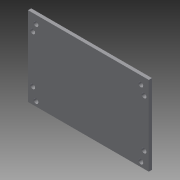
# Autodesk Inventor part: circuit_plate
Saved by Autodesk Inventor 2013 (Build 170138000, 138)
## iProperties
Created: 2014-05-23
Part Number: circuit_plate
Material: 一般
Document SubType Name: Modeling
Designer: andou
Density: 1 g/cm^3
Author: andou
Autodesk Inventor part; units mm, degrees
ref_plane "YZ Plane" through (0, 0, 0) normal (1, 0, 0) x (0, 1, 0)
ref_plane "XZ Plane" through (0, 0, 0) normal (0, 1, 0) x (-1, 0, 0)
ref_plane "XY Plane" through (0, 0, 0) normal (0, 0, 1) x (1, 0, 0)
sketch "スケッチ1" plane through (0, 0, 0) normal (0, 1, 0) x (-1, 0, 0)
  line L0 (-38, 35) -> (38, 35)
  line L1 (38, 35) -> (38, -15)
  line L2 (38, -15) -> (-38, -15)
  line L3 (-38, -15) -> (-38, 35)
  point P0 (0, 0)
  dimension "d0" = 76
  dimension "d3" = 50
  dimension "d4" = 35
  dimension "d5" = 38
  constraints: 8 end point, 2 parallel, 1 horizontal, 1 perpendicular
  measures "d0" distance of L0.start L0.end
  measures "d3" distance of L2.end L0.start
  measures "d4" distance from line of L0 point (0, 0)
  measures "d5" distance from line of L3 point (0, 0)
extrude "押し出し1" add sketch "スケッチ1" along normal blind 2
sketch "スケッチ2" plane through (0, 2, 0) normal (0, 1, 0) x (1, 0, 0)
  line L0 (-38, -35) -> (38, -35) projected
  line L1 (38, -35) -> (38, 15) projected
  line L2 (38, 15) -> (-38, 15) projected
  line L3 (-38, 15) -> (-38, -35) projected
  circle A0 centre (-35, 5) radius 1.5
  circle A1 centre (-35, -25) radius 1.5
  circle A2 centre (35, -25) radius 1.5
  circle A3 centre (35, 5) radius 1.5
  point P0 (0, 0)
  dimension "d9" = 3
  dimension "d10" = 30
  dimension "d11" = 70
  dimension "d12" = 70
  dimension "d13" = 3
  dimension "d14" = 10
  dimension "d15" = 30
  dimension "d16" = 3
  dimension "d19" = 10
  constraints: 4 centre point, 3 equal radius
  measures "d9" distance from line of L3 A0.centre
  measures "d10" distance of A1.centre A0.centre
  measures "d11" distance of A3.centre A0.centre
  measures "d12" distance of A2.centre A1.centre
  measures "d13" distance from line of L3 A1.centre
  measures "d14" distance from line of L0 A2.centre
  measures "d15" distance of A3.centre A2.centre
  measures "d16" diameter of A3
  measures "d19" distance from line of A1.centre L0
extrude "押し出し2" cut sketch "スケッチ2" against normal blind 2 keep common part
sketch "スケッチ3" plane through (0, 2, 0) normal (0, 1, 0) x (1, 0, 0)
  circle A0 centre (35, 5) radius 1.5 projected
  circle A1 centre (35, -25) radius 1.5 projected
  circle A2 centre (-35, -25) radius 1.5 projected
  circle A3 centre (-35, 5) radius 1.5 projected
  line L0 (-38, -35) -> (38, -35) projected
  line L1 (38, -35) -> (38, 15) projected
  line L2 (38, 15) -> (-38, 15) projected
  line L3 (-38, 15) -> (-38, -35) projected
  circle A4 centre (-33, 12) radius 1.5
  circle A5 centre (-33, -30) radius 1.5
  circle A6 centre (33, -30) radius 1.5
  circle A7 centre (33, 12) radius 1.5
  point P0 (0, 0)
  dimension "d20" = 66
  dimension "d22" = 42
  dimension "d23" = 42
  dimension "d24" = 66
  dimension "d25" = 5
  dimension "d26" = 5
  dimension "d27" = 5
  dimension "d28" = 5
  constraints: 4 centre point, 4 equal radius
  measures "d20" distance of A7.centre A4.centre
  measures "d22" distance of A4.centre A5.centre
  measures "d23" distance of A6.centre A7.centre
  measures "d24" distance of A6.centre A5.centre
  measures "d25" distance from line of L0 A5.centre
  measures "d26" distance from line of A6.centre L0
  measures "d27" distance from line of L3 A5.centre
  measures "d28" distance from line of L3 A4.centre
extrude "押し出し3" cut sketch "スケッチ3" against normal blind 2 keep common part
